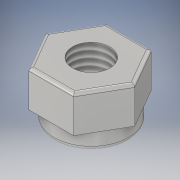
# Autodesk Inventor part: Tuerca_chica
Saved by Autodesk Inventor 2019 (Build 230136000, 136)
## iProperties
Created: 2019-09-23
Part Number: Tuerca_chica
Material: Genérico
Document SubType Name: Modeling
Designer: axelj
Density: 1 g/cm^3
Appearance: Aluminio - Pulido
Author: axelj
Autodesk Inventor part; units mm, degrees
ref_plane "YZ Plane" through (0, 0, 0) normal (1, 0, 0) x (0, 1, 0)
ref_plane "XZ Plane" through (0, 0, 0) normal (0, 1, 0) x (-1, 0, 0)
ref_plane "XY Plane" through (0, 0, 0) normal (0, 0, 1) x (1, 0, 0)
sketch "Boceto1" plane through (0, 0, 0) normal (0, 1, 0) x (-1, 0, 0)
  circle A0 centre (0, 0) radius 1.25
  line L0 (-3, 0.0868) -> (-1.5, -2.5112)
  line L1 (-3, 0.0868) -> (0, 0.0868) construction
  line L2 (-1.5, -2.5112) -> (1.5, -2.5112)
  line L3 (1.5, -2.5112) -> (3, 0.0868)
  line L4 (1.5, -2.5112) -> (4.5, -2.5112) construction
  line L5 (-3, 0.0868) -> (-1.5, 2.6849)
  line L6 (-1.5, 2.6849) -> (1.5, 2.6849)
  line L7 (1.5, 2.6849) -> (3, 0.0868)
  point P0 (0, 0)
  dimension "d1" = 2.5
  dimension "d8" = 3
  dimension "d9" = 60
  dimension "d10" = 3
  dimension "d12" = 3
  dimension "d14" = 120
  dimension "d15" = 120
  dimension "d16" = 3
  dimension "d17" = 3
  constraints: 16 end point, 3 horizontal, 2 equal length, 1 centre point
  measures "d1" diameter of A0
  measures "d8" distance of L0.start L0.end
  measures "d9" angle of L0 L1
  measures "d10" distance of L0.end L2.end
  measures "d12" distance of L2.end L3.end
  measures "d14" angle of L2 L0
  measures "d15" angle of L3 L2
  measures "d16" horizontal distance of L3.end A0.centre
  measures "d17" horizontal distance of point (0, 0) L0.start
extrude "Extrusión2" add sketch "Boceto1" along normal blind 2.5
sketch "Boceto3" plane through (0, 0, 0) normal (0, -1, 0) x (1, 0, 0)
  circle A0 centre (0, 0) radius 2.5
  circle A1 centre (0, 0) radius 1.25
  dimension "d20" = 5
  dimension "d21" = 2.5
  constraints: 2 centre point, 2 coincident
  measures "d20" diameter of A0
  measures "d21" diameter of A1
extrude "Extrusión3" add sketch "Boceto3" along normal blind 1.2
fillet "Empalme2" radius 0.3 1 edges at (-2.5, -1.2, 0)
fillet "Empalme3" radius 0.02 1 edges at (-2.5, 0, 0)
fillet "Empalme4" radius 0.05 8 edges at (0, 0, -2.5112) (-0.8551, 0, -2.5112) (0.8551, 0, -2.5112) (2.25, 0, -1.2122) (2.25, 0, 1.3859) (0, 0, 2.6849) (-2.25, 0, 1.3859) (-2.25, 0, -1.2122)
fillet "Empalme5" radius 0.2 6 edges at (-2.25, 2.5, -1.2122) (0, 2.5, -2.5112) (2.25, 2.5, -1.2122) (-2.25, 2.5, 1.3859) (0, 2.5, 2.6849) (2.25, 2.5, 1.3859)
thread "Rosca1" size "M2.5x0.45" class "6H" standard "ANSI Metric M Profile" full length
